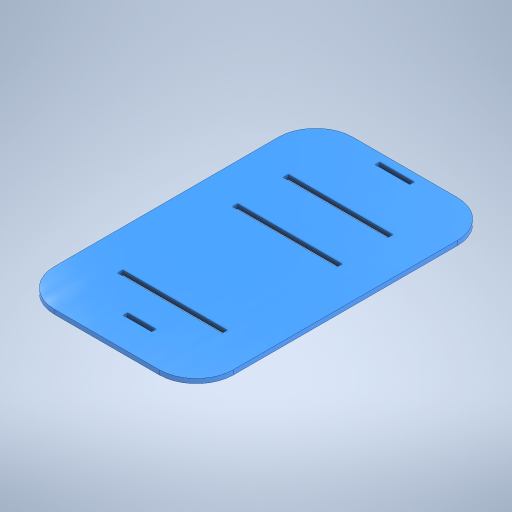
# Autodesk Inventor part: Base1
Saved by Autodesk Inventor 2024.3 (Build 283343000, 343)
## iProperties
Created: 2024-05-14
Part Number: Base1
Material: PMMA Plastic
Document SubType Name: Modeling
Designer: USUARIO
Mass: 48.8268 g
Surface Area: 294.76 cm^2
Volume: 41.1 cm^3
Density: 1.188 g/cm^3
Appearance: Cyan
Author: USUARIO
Autodesk Inventor part; units mm, degrees
ref_plane "YZ Plane" through (0, 0, 0) normal (1, 0, 0) x (0, 1, 0)
ref_plane "XZ Plane" through (0, 0, 0) normal (0, 1, 0) x (-1, 0, 0)
ref_plane "XY Plane" through (0, 0, 0) normal (0, 0, 1) x (1, 0, 0)
sketch "Sketch1" plane through (0, 0, 0) normal (0, 1, 0) x (-1, 0, 0)
  line L0 (25, 0) -> (95, 0)
  line L1 (120, -25) -> (120, -130)
  line L2 (120, -130) -> (0, -130) construction
  line L3 (0, -130) -> (0, -25)
  line L4 (0, -77.5) -> (25, -77.5) construction
  line L5 (25, -77.5) -> (25, -45.5) construction
  line L6 (25, -45.5) -> (25, -42.5)
  line L7 (25, -42.5) -> (95, -42.5) construction
  line L8 (95, -42.5) -> (95, -45.5)
  line L9 (95, -45.5) -> (25, -45.5) construction
  line L10 (25, -77.5) -> (25, -119.5) construction
  line L11 (25, -119.5) -> (25, -122.5)
  line L12 (25, -122.5) -> (95, -122.5) construction
  line L13 (95, -122.5) -> (95, -119.5)
  line L14 (95, -119.5) -> (25, -119.5) construction
  line L15 (0, -130) -> (120, -130) construction
  line L16 (120, -130) -> (120, -175)
  line L17 (95, -200) -> (25, -200)
  line L18 (0, -175) -> (0, -130)
  line L19 (25, -122.5) -> (25, -156.5) construction
  line L20 (25, -156.5) -> (95, -156.5) construction
  line L21 (95, -156.5) -> (95, -130) construction
  line L22 (95, -130) -> (25, -130) construction
  line L23 (25, -130) -> (25, -156.5) construction
  line L24 (60, -156.5) -> (60, -191.5) construction
  line L25 (60, -191.5) -> (48.5, -191.5) construction
  line L26 (48.5, -191.5) -> (48.5, -194.5) construction
  line L27 (48.5, -194.5) -> (60, -194.5) construction
  line L28 (60, -194.5) -> (60, -191.5) construction
  line L29 (48.5, -191.5) -> (71.5, -191.5)
  line L30 (71.5, -191.5) -> (71.5, -194.5)
  line L31 (71.5, -194.5) -> (48.5, -194.5)
  line L32 (48.5, -194.5) -> (48.5, -191.5)
  line L33 (25, -156.5) -> (95, -156.5) construction
  line L34 (95, -156.5) -> (95, -153.5)
  line L35 (95, -153.5) -> (25, -153.5) construction
  line L36 (25, -153.5) -> (25, -156.5)
  line L37 (60, -42.5) -> (60, -22.5) construction
  line L38 (60, -22.5) -> (68.5, -22.5) construction
  line L39 (68.5, -22.5) -> (49.5, -22.5)
  line L40 (49.5, -22.5) -> (49.5, -19.5)
  line L41 (49.5, -19.5) -> (68.5, -19.5)
  line L42 (68.5, -19.5) -> (68.5, -22.5)
  line L43 (95, -42.5) -> (95, -42.25)
  line L44 (95, -42.25) -> (25, -42.25)
  line L45 (25, -42.25) -> (25, -42.5)
  line L46 (95, -45.5) -> (95, -45.75)
  line L47 (95, -45.75) -> (25, -45.75)
  line L48 (25, -45.75) -> (25, -45.5)
  line L49 (95, -119.5) -> (95, -119.25)
  line L50 (95, -119.25) -> (25, -119.25)
  line L51 (25, -119.25) -> (25, -119.5)
  line L52 (95, -122.5) -> (95, -122.75)
  line L53 (95, -122.75) -> (25, -122.75)
  line L54 (25, -122.75) -> (25, -122.5)
  line L55 (95, -156.5) -> (95, -156.75)
  line L56 (95, -156.75) -> (25, -156.75)
  line L57 (25, -156.75) -> (25, -156.5)
  line L58 (25, -153.5) -> (25, -153.25)
  line L59 (25, -153.25) -> (95, -153.25)
  line L60 (95, -153.25) -> (95, -153.5)
  arc A0 (95, -200) -> (120, -175) centre (95, -175) ccw
  arc A1 (0, -175) -> (25, -200) centre (25, -175) ccw
  arc A2 (25, 0) -> (0, -25) centre (25, -25) ccw
  arc A3 (120, -25) -> (95, 0) centre (95, -25) ccw
  point P0 (0, 0)
  point P1 (120, 0)
  point P2 (120, -200)
  point P3 (0, -200)
  point P4 (100, -120)
  point P5 (100, -120)
  point P6 (25, -153.5)
  dimension "d0" = 120
  dimension "d1" = 130
  dimension "d2" = 25
  dimension "d3" = 32
  dimension "d4" = 3
  dimension "d5" = 70
  dimension "d6" = 42
  dimension "d7" = 3
  dimension "d8" = 70
  dimension "d11" = 70
  dimension "d12" = 34
  dimension "d14" = 35
  dimension "d15" = 11.5
  dimension "d16" = 3
  dimension "d17" = 23
  dimension "d18" = 3
  dimension "d19" = 70
  dimension "d20" = 3
  dimension "d24" = 20
  dimension "d25" = 8.5
  dimension "d26" = 19
  dimension "d27" = 3
  dimension "d28" = 70
  dimension "d29" = 0.25
  dimension "d30" = 70
  dimension "d31" = 0.25
  dimension "d32" = 0.25
  dimension "d33" = 70
  dimension "d34" = 0.25
  dimension "d35" = 0.25
  dimension "d36" = 70
  dimension "d37" = 0.25
  dimension "d38" = 0.25
  dimension "d39" = 70
  dimension "d40" = 0.25
  dimension "d41" = 0.25
  dimension "d42" = 70
  dimension "d43" = 0.25
  dimension "d44" = 0.25
  dimension "d45" = 70
  dimension "d46" = 0.25
  dimension "d47" = 25
  dimension "d48" = 25
  constraints: 122 end point, 19 point on line, 15 perpendicular, 14 parallel, 9 horizontal, 8 point on circle, 8 tangent, 8 vertical, 4 centre point, 3 midpoint, 2 collinear, 2 equal radius
  measures "d0" distance of L1.end L2.end
  measures "d1" distance of point (120, 0) L1.end
  measures "d2" distance of L4.start L4.end
  measures "d3" distance of L4.end L5.end
  measures "d4" distance of L5.end L6.end
  measures "d5" distance of L6.end L7.end
  measures "d6" distance of L4.end L10.end
  measures "d7" distance of L10.end L11.end
  measures "d8" distance of L11.end L12.end
  measures "d11" distance of L1.end point (120, -200)
  measures "d12" distance of L11.end L19.end
  measures "d14" distance of L24.start L24.end
  measures "d15" distance of L27.end L26.end
  measures "d16" distance of L26.end L25.end
  measures "d17" distance of L30.end L31.end
  measures "d18" distance of L29.end L30.end
  measures "d19" distance of L35.end L34.end
  measures "d20" distance of L34.end L33.end
  measures "d24" distance of L37.start L37.end
  measures "d25" distance of L37.end L38.end
  measures "d26" distance of L40.end L41.end
  measures "d27" distance of L39.end L40.end
  measures "d28" distance of L21.end L22.end
  measures "d29" distance of L7.end L43.end
  measures "d30" distance of L43.end L44.end
  measures "d31" distance of L44.end L6.end
  measures "d32" distance of L8.end L46.end
  measures "d33" distance of L46.end L47.end
  measures "d34" distance of L47.end L5.end
  measures "d35" distance of L13.end L49.end
  measures "d36" distance of L49.end L50.end
  measures "d37" distance of L50.end L10.end
  measures "d38" distance of L12.end L52.end
  measures "d39" distance of L52.end L53.end
  measures "d40" distance of L53.end L11.end
  measures "d41" distance of L33.end L55.end
  measures "d42" distance of L55.end L56.end
  measures "d43" distance of L56.end L19.end
  measures "d44" distance of L35.end L58.end
  measures "d45" distance of L58.end L59.end
  measures "d46" distance of L59.end L34.end
  measures "d47" radius of A0
  measures "d48" radius of A1
extrude "Extrusion1" add sketch "Sketch1" along normal blind 3
body "Solid1"
